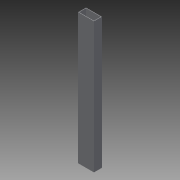
# Autodesk Inventor part: WG18 waveguide
Saved by Autodesk Inventor 2015 (Build 190159000, 159)
## iProperties
Created: 2014-05-20
Part Number: WG18 waveguide
Material: Generic
Document SubType Name: Modeling
Designer: jad211
Density: 1 g/cm^3
Appearance: Default
Author: jad211
Autodesk Inventor part; units mm, degrees
ref_plane "YZ Plane" through (0, 0, 0) normal (1, 0, 0) x (0, 1, 0)
ref_plane "XZ Plane" through (0, 0, 0) normal (0, 1, 0) x (-1, 0, 0)
ref_plane "XY Plane" through (0, 0, 0) normal (0, 0, 1) x (1, 0, 0)
sketch "Sketch1" plane through (0, 0, 0) normal (0, 1, 0) x (-1, 0, 0)
  line L0 (0, 0) -> (15.799, 0)
  line L1 (15.799, 0) -> (15.799, -7.899)
  line L2 (15.799, -7.899) -> (0, -7.899)
  line L3 (0, -7.899) -> (0, 0)
  line L4 (0.5, -0.5) -> (15.299, -0.5)
  line L5 (15.299, -0.5) -> (15.299, -7.399)
  line L6 (15.299, -7.399) -> (0.5, -7.399)
  line L7 (0.5, -7.399) -> (0.5, -0.5)
  dimension "d0" = 15.799
  dimension "d1" = 7.899
  dimension "d2" = 0.5
  dimension "d3" = 0.5
  dimension "d4" = 0.5
  dimension "d5" = 0.5
  constraints: 16 end point
  measures "d0" distance of L1.end L2.end
  measures "d1" distance of L0.end L1.end
  measures "d2" distance between parallel lines of L3 L7
  measures "d3" distance between parallel lines of L1 L5
  measures "d4" distance between parallel lines of L0 L4
  measures "d5" distance between parallel lines of L2 L6
extrude "Extrusion1" add sketch "Sketch1" along normal blind 131
body "Solid1"
